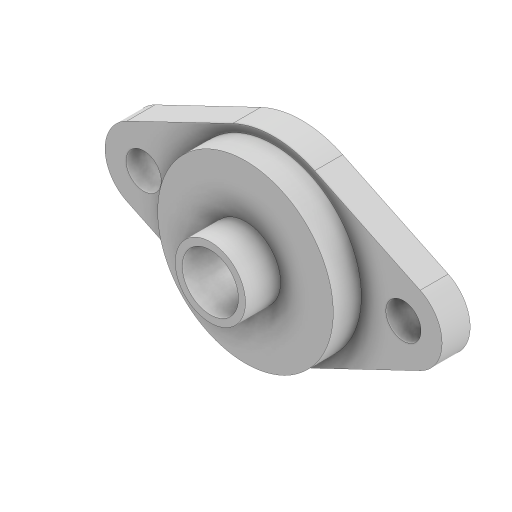
# Autodesk Inventor part: RODAMIENTO DE PARED
Saved by Autodesk Inventor 2024 (Build 280153000, 153)
## iProperties
Created: 2024-06-28
Part Number: RODAMIENTO DE PARED
Material: Generic
Document SubType Name: Modeling
Designer: Jhuliams
Density: 1 g/cm^3
Appearance: Default
Author: Jhuliams
Autodesk Inventor part; units mm, degrees
ref_plane "YZ Plane" through (0, 0, 0) normal (1, 0, 0) x (0, 1, 0)
ref_plane "XZ Plane" through (0, 0, 0) normal (0, 1, 0) x (-1, 0, 0)
ref_plane "XY Plane" through (0, 0, 0) normal (0, 0, 1) x (1, 0, 0)
sketch "Sketch1" plane through (0, 0, 0) normal (0, 0, 1) x (1, 0, 0)
  line L0 (0, 0) -> (-18.5, 0)
  circle A0 centre (-18.5, 0) radius 2.5
  line L1 (-20.8784, 4.9592) -> (-5.8378, 12.1725)
  line L2 (-20.8784, -4.9592) -> (-5.8378, -12.1725)
  arc A1 (-20.8784, 4.9592) -> (-20.8784, -4.9592) centre (-18.5, 0) ccw
  line L3 (0, 0) -> (0, 5.7402)
  circle A2 centre (18.5, 0) radius 2.5
  line L4 (20.8784, 4.9592) -> (5.8378, 12.1725)
  line L5 (20.8784, -4.9592) -> (5.8378, -12.1725)
  arc A3 (20.8784, -4.9592) -> (20.8784, 4.9592) centre (18.5, 0) ccw
  arc A4 (-5.8378, -12.1725) -> (5.8378, -12.1725) centre (0, 0) ccw
  arc A5 (5.8378, 12.1725) -> (-5.8378, 12.1725) centre (0, 0) ccw
  point P0 (10.0991, 19.8157)
  point P1 (10.0991, -19.8157)
  dimension "d1" = 18.5
  dimension "d2" = 5
  constraints: 12 end point, 8 point on circle, 8 symmetric about line, 6 centre point, 5 coincident, 2 tangent, 1 horizontal, 1 vertical, 2 other
  measures "d1" distance of L0.start L0.end
  measures "d2" diameter of A0
extrude "Extrusion1" add sketch "Sketch1" along normal blind 4
sketch "Sketch2" plane through (0, 0, 4) normal (0, 0, 1) x (1, 0, 0)
  circle A0 centre (0, 0) radius 12.5
  dimension "d6" = 25
  constraints: 1 centre point, 1 coincident
  measures "d6" diameter of A0
extrude "Extrusion2" add sketch "Sketch2" along normal blind 4
sketch "Sketch3" plane through (0, 0, 8) normal (0, 0, 1) x (1, 0, 0)
  circle A0 centre (0, 0) radius 4
  circle A1 centre (0, 0) radius 5
  dimension "d9" = 8
  dimension "d10" = 10
  constraints: 2 centre point, 2 coincident
  measures "d9" diameter of A0
  measures "d10" diameter of A1
extrude "Extrusion3" add sketch "Sketch3" along normal blind 5
sketch "Sketch4" plane through (0, 0, 8) normal (0, 0, 1) x (1, 0, 0)
  circle A0 centre (0, 0) radius 4 projected
extrude "Extrusion4" cut sketch "Sketch4" against normal blind 10
body "Solid1"
